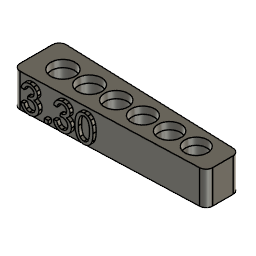
HoleDiaTest3.3mm_v7 (Autodesk Fusion 360 design; units mm, degrees)
Autodesk Fusion 360 part; units mm, degrees
sketch "Sketch1" plane through (0, 0, 0) normal (0, 0, 1) x (1, 0, 0)
  circle A0 centre (0, 0) radius 1.65
  circle A1 centre (4, 0) radius 1.625
  circle A2 centre (8, 0) radius 1.6
  circle A3 centre (-4, 0) radius 1.675
  circle A4 centre (-8, 0) radius 1.7
  circle A5 centre (-12, 0) radius 1.725
  line L0 (-12, 0) -> (8, 0) construction
  line L1 (8, 0) -> (7.5, 0) construction
  line L2 (-12, 0) -> (-16, 0) construction
  line L3 (8, 0) -> (12, 0) construction
  line L4 (-16, -3.5) -> (-16, 3.5)
  line L5 (12, -2.5) -> (12, 2.5)
  line L6 (12, 2.5) -> (-16, 3.5)
  line L7 (-16, -3.5) -> (12, -2.5)
  dimension "d1" = 3.3
  dimension "d2" = 3.25
  dimension "d3" = 3.2
  dimension "d4" = 3.35
  dimension "d5" = 3.4
  dimension "d6" = 3.45
  dimension "d7" = 4
  dimension "d8" = 4
  dimension "d10" = 4
  dimension "d11" = 4
  dimension "d25" = 4
  dimension "d29" = 4
  dimension "d30" = 4
  constraint coincident A5.centre L0.start
  constraint coincident A2.centre L0.end
  constraint parallel L0 L1
  constraint parallel L0 L2
  constraint parallel L0 L3
  constraint midpoint L2.end L4
  constraint perpendicular L2 L4
  constraint midpoint L3.end L5
  constraint perpendicular L3 L5
  measures "d1" diameter of A0
  measures "d2" diameter of A1
  measures "d3" diameter of A2
  measures "d4" diameter of A3
  measures "d5" diameter of A4
  measures "d6" diameter of A5
  measures "d7" distance of A4.centre A5.centre
  measures "d8" distance of A3.centre A4.centre
  measures "d10" distance of A0.centre A1.centre
  measures "d11" distance of A1.centre A2.centre
  measures "d25" distance of A0.centre A3.centre
  measures "d29" distance of A5.centre L2.end
  measures "d30" distance of A2.centre L3.end
extrude "Extrude1" add sketch "Sketch1" against normal blind 5
fillet "Fillet2" radius 1 4 edges at (-16, 3.5, -2.5) (-16, -3.5, -2.5) (12, 2.5, -2.5) (12, -2.5, -2.5)
chamfer "Chamfer2" distance 0.1 distance2 1 6 edges at (-13.6083, -0.6238, -5) (-9.585, -0.6147, -5) (-5.5616, -0.6057, -5) (-1.5383, -0.5967, -5) (2.485, -0.5876, -5) (6.5083, -0.5786, -5) measured on face at (-15.2417, 0, -5) measured on face at (-15.2417, 0, -5) measured on face at (-15.2417, 0, -5) measured on face at (-15.2417, 0, -5) measured on face at (-15.2417, 0, -5) measured on face at (-15.2417, 0, -5) tangent chain off
chamfer "Chamfer3" distance 1 distance2 0.1 6 edges at (-13.6083, -0.6238, 0) (-9.585, -0.6147, 0) (-5.5616, -0.6057, 0) (-1.5383, -0.5967, 0) (2.485, -0.5876, 0) (6.5083, -0.5786, 0) measured on face at (-10.2771, -0.086, -2.6667) measured on face at (-6.3021, -0.0847, -2.6667) measured on face at (-2.3271, -0.0835, -2.6667) measured on face at (1.6479, -0.0822, -2.6667) measured on face at (5.623, -0.081, -2.6667) measured on face at (9.598, -0.0798, -2.6667) tangent chain off
sketch "Sketch2" plane through (0.1045, -2.9248, 0) normal (0.035692, -0.999363, 0) x (0.999363, 0.035692, 0)
  line L0 (10.9382, -5) -> (10.9382, 0)
  line L1 (10.9382, 0) -> (-15.0784, 0)
  line L2 (-15.0784, 0) -> (-15.0784, -5)
  line L3 (-15.0784, -5) -> (10.9382, -5)
  line L4 (-14.5, -4.5) -> (7.5, -4.5) construction
  line L5 (7.5, -4.5) -> (7.5, -0.5) construction
  line L6 (7.5, -0.5) -> (-14.5, -0.5) construction
  line L7 (-14.5, -0.5) -> (-14.5, -4.5) construction
  dimension "d37" = 4
  dimension "d38" = 0
  text T0 "3.30" font "Arial" height 4 align left top in box 22 x 4 at (-14.5, -4.5) x (1, 0) y (0, 1) spacing 1.01 kerned
extrude "Extrude3" add sketch "Sketch2" along normal blind 0.5 text T0
equation "d38 = '3.30'"
